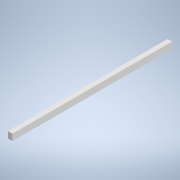
# Autodesk Inventor part: support_rod_right
Saved by Autodesk Inventor 2021 (Build 250183000, 183)
## iProperties
Created: 2021-06-26
Part Number: support_rod_right
Material: Generic
Document SubType Name: Modeling
Designer: TARUN
Density: 1 g/cm^3
Appearance: Default
Author: TARUN
Autodesk Inventor part; units mm, degrees
ref_plane "YZ Plane" through (0, 0, 0) normal (1, 0, 0) x (0, 1, 0)
ref_plane "XZ Plane" through (0, 0, 0) normal (0, 1, 0) x (-1, 0, 0)
ref_plane "XY Plane" through (0, 0, 0) normal (0, 0, 1) x (1, 0, 0)
sketch "Sketch1" plane through (0, 0, 0) normal (0, 0, 1) x (1, 0, 0)
  line L0 (-3.5, -5) -> (3.5, -5)
  line L1 (3.5, -5) -> (3.5, 5)
  line L2 (3.5, 5) -> (-3.5, 5)
  line L3 (-3.5, 5) -> (-3.5, -5)
  line L4 (-3.5, -5) -> (3.5, 5) construction
  line L5 (3.5, -5) -> (-3.5, 5) construction
  point P0 (0, 0)
  dimension "d0" = 7
  dimension "d1" = 10
  constraints: 12 end point, 2 midpoint, 2 parallel, 1 horizontal, 1 perpendicular
  measures "d0" distance of L2.end L1.end
  measures "d1" distance of L1.end L0.end
extrude "Extrusion1" add sketch "Sketch1" along normal blind 250
sketch "Sketch2" plane through (-3.5, -5, 0) normal (-1, 0, 0) x (0, 0, 1)
  line L0 (0, 0) -> (250, 0) projected
  line L1 (0, 10) -> (250, 10) projected
  line L2 (65, 0) -> (70, 0)
  line L3 (70, 0) -> (70, 10)
  line L4 (70, 10) -> (65, 10)
  line L5 (65, 10) -> (65, 0)
  point P0 (0, 5)
  dimension "d4" = 5
  dimension "d5" = 65
  constraints: 8 end point, 2 parallel, 2 point on line, 1 horizontal, 1 perpendicular
  measures "d4" distance of L4.end L3.end
  measures "d5" distance from line of L5 point (0, 5)
extrude "Extrusion2" add sketch "Sketch2" along normal blind 100
fillet "Fillet1" radius 2 2 edges at (-103.5, 0, 65) (-103.5, 0, 70)
sketch "Sketch3" plane through (3.5, 5, 250) normal (0, 1, 0) x (1, 0, 0)
  circle A0 centre (-103.2335, 182.6391) radius 2
  point P0 (-3.5, 250)
  dimension "d9" = 4
  constraints: 1 centre point
  measures "d9" diameter of A0
extrude "Extrusion3" cut sketch "Sketch3" against normal through all
body "Solid1"
